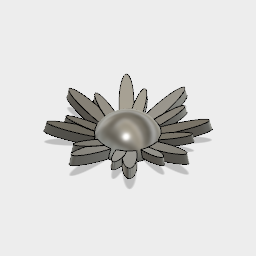
xiaoFA v1 (Autodesk Fusion 360 design; units mm, degrees)
Autodesk Fusion 360 part; units mm, degrees
sketch "草图1" plane through (0, 0, 0) normal (0, 1, 0) x (1, 0, 0)
  ellipse E0 centre (-11.2867, 8.0478) end of major axis (-1.2867, 8.0478) minor radius 2
  line L0 (-21.2867, 8.0478) -> (-1.2867, 8.0478)
  line L1 (-11.2867, 6.0478) -> (-11.2867, 10.0478)
extrude "拉伸1" add sketch "草图1" along normal blind 3 makes body 1
move_body "移动1" bodies 1 to x (1, 0, 0) y (0, 1, 0) z (0, 0, 1) at (0, 0, 15)
move_body "移动2" bodies 1 to x (0.965926, 0.258819, 0) y (-0.258819, 0.965926, 0) z (0, 0, 1) at (-0.7253, 5.5094, 0)
move_body "移动3" bodies 1 to x (1, 0, 0) y (0, 1, 0) z (0, 0, 1) at (0, 0, -10)
box "长方体基本要素1" add length 8.8241 width 7.865 height 5 placed x (0, 0, 1) y (1, 0, 0) z (0, 1, 0) at (-39.9003, 0, -7.3854) separate body makes body 2
move_body "移动4" bodies 2 to x (1, 0, 0) y (0, 1, 0) z (0, 0, 1) at (5.7549, 0, -0.1918)
move_face "MoveFace1" by (-0.6043, 0.3699, -0.7656) 1 faces at (-28.9022, 5, -4.6359) on bodies 2
move_face "MoveFace2" by (-2.4598, 0.5548, 1.9049) 1 faces at (-26.2805, 1.79, -1.6945) on bodies 2
move_face "MoveFace3" by (2.2682, 1.1097, -3.3779) 1 faces at (-32.3438, 1.79, 1.2469) on bodies 2
move_face "MoveFace4" by (0.8252, -1.4102, 0.585) 1 faces at (-30.542, 5.3699, -5.7618) on bodies 2
move_face "MoveFace5" by (0.7137, 0.2543, -0.9681) 1 faces at (-32.3438, 1.3199, -2.131) on bodies 2
move_face "MoveFace6" by (-1.4818, 0.6011, 0.8807) 1 faces at (-28.7403, 1.3199, -4.5918) on bodies 2
move_body "移动5" bodies 2 to x (1, 0, 0) y (0, 1, 0) z (0, 0, 1) at (2.1471, -2.6124, 0.4653)
move_body "移动6" bodies 2 to x (1, 0, 0) y (0, 1, 0) z (0, 0, 1) at (3.6769, 2.6021, 0)
pattern_circular "C-阵列1" count 8 over 360 about axis through (-24.398, 3.9494, -2.6337) along (0, -1, 0) of bodies 1 makes body 3 at (-13.7959, 3.2332, 8.2287) makes body 4 at (-23.3859, 4.841, 6.9532) makes body 5 at (-34.7114, 6.131, 7.4194) makes body 6 at (-34.7614, 1.9432, -1.6216) makes body 7 at (-35.0002, 3.2332, -13.4962) makes body 8 at (-24.214, 6.131, -17.035) makes body 9 at (-17.7857, 1.9432, -10.6774)
copy_body "复制和粘贴实体1" bodies 1 4 8 5 7 6 3 9 makes body 10 makes body 11 makes body 12 makes body 13 makes body 14 makes body 15 makes body 16 makes body 17
scale "缩放1" factor 0.8 about (-22.0632, 2.8978, -3.0478) bodies 17 16 15 14 13 12 11 10
move_body "移动7" bodies 10 12 16 13 15 17 14 11 to x (0.965926, 0, 0.258819) y (0, 1, 0) z (-0.258819, 0, 0.965926) at (-1.513, 0, 6.2249)
sphere "球体基本要素1" add diameter 20 placed x (1, 0, 0) y (0, 0, -1) z (0, 1, 0) at (-24.3685, 0, -2.5234) bodies 1 3 4 5 6 7 8 9 10 11 12 13 14 15 16 17
move_body "移动8" bodies 2 to x (1, 0, 0) y (0, 1, 0) z (0, 0, 1) at (0.0632, -2.9686, 0)
move_face "MoveFace7" by (5.8, 0, 0) 1 faces at (-24.3349, -1.659, -4.1265) on bodies 2
move_face "MoveFace8" by (0, 0, 4.8) 1 faces at (-25.0172, -1.659, -2.6337) on bodies 2
move_face "MoveFace9" by (0, 0, -4) 1 faces at (-25.0172, -1.659, -7.1119) on bodies 2
move_face "MoveFace10" by (-29, 0, 0) 1 faces at (-28.2583, -1.659, -2.2598) on bodies 2
move_face "MoveFace11" by (0, 0, 20) 1 faces at (-31.4427, -1.659, 2.1663) on bodies 2
move_face "MoveFace12" by (31, 0, 0) 1 faces at (-18.5349, -1.659, 11.0735) on bodies 2
move_face "MoveFace13" by (0, 0, -27) 1 faces at (-34.0172, -1.659, -11.1119) on bodies 2
move_body "移动9" bodies 1 to x (1, 0, 0) y (0, 1, 0) z (0, 0, 1) at (2.9454, 0, 4.0557)
move_body "移动10" bodies 1 to x (1, 0, 0) y (0, 1, 0) z (0, 0, 1) at (-0.1033, -0.6994, -0.2431)
move_face "MoveFace14" by (0.1711, -5.4534, 1.1784) 1 faces at (-34.0172, -1.659, 22.1663) on bodies 2
move_face "MoveFace15" by (1.1603, -0.893, -0.2674) 1 faces at (-34.0172, -1.659, 23.3447) on bodies 2
move_face "MoveFace16" by (0.3231, -9.2574, -3.4545) 1 faces at (-10.776, -2.9789, -17.7155) on bodies 2
combine "合并1" operation cut target body 1 tool bodies 2
